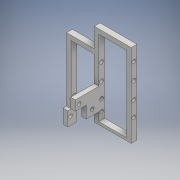
# Autodesk Inventor part: Mounting bracket
Saved by Autodesk Inventor 2017 (Build 210142000, 142)
## iProperties
Created: 2018-11-02
Part Number: Mounting bracket
Material: Generic
Document SubType Name: Modeling
Designer: Usman
Density: 1 g/cm^3
Appearance: Default
Author: Usman
Autodesk Inventor part; units mm, degrees
ref_plane "YZ Plane" through (0, 0, 0) normal (1, 0, 0) x (0, 1, 0)
ref_plane "XZ Plane" through (0, 0, 0) normal (0, 1, 0) x (-1, 0, 0)
ref_plane "XY Plane" through (0, 0, 0) normal (0, 0, 1) x (1, 0, 0)
sketch "Sketch1" plane through (0, 0, 0) normal (0, 1, 0) x (-1, 0, 0)
  line L0 (0, 0) -> (-30, 0)
  line L1 (-30, 0) -> (-30, -80)
  line L2 (0, 0) -> (0, -21)
  line L3 (0, -21) -> (30, -21)
  line L4 (30, -21) -> (30, -80)
  line L5 (30, -80) -> (30, -112)
  line L6 (30, -112) -> (8.74, -112)
  line L7 (8.74, -112) -> (8.74, -80)
  line L8 (8.74, -80) -> (-30, -80)
  line L9 (-35, 5) -> (-35, -85)
  line L10 (-35, -85) -> (3.74, -85)
  line L11 (3.74, -85) -> (3.74, -117)
  line L12 (-35, 5) -> (5, 5)
  line L13 (5, 5) -> (5, -16)
  line L14 (5, -16) -> (35, -16)
  line L15 (35, -16) -> (35, -117)
  line L16 (35, -117) -> (3.74, -117)
  line L17 (0, -21) -> (5, -21)
  line L18 (0, -21) -> (5, -21)
  line L19 (5, -21) -> (5, -80)
  line L20 (0, -21) -> (0, -80)
  dimension "d0" = 30
  dimension "d2" = 21
  dimension "d3" = 30
  dimension "d4" = 59
  dimension "d5" = 32
  dimension "d6" = 21.26
  dimension "d9" = 90
  dimension "d10" = 38.74
  dimension "d11" = 32
  dimension "d12" = 40
  dimension "d13" = 21
  dimension "d14" = 30
  constraints: 42 end point, 13 perpendicular, 4 point on line, 2 horizontal, 2 vertical, 1 collinear, 1 parallel
  measures "d0" distance of L0.start L0.end
  measures "d2" distance of L0.start L2.end
  measures "d3" distance of L2.end L3.end
  measures "d4" distance of L3.end L4.end
  measures "d5" distance of L4.end L5.end
  measures "d6" distance of L5.end L6.end
  measures "d9" distance of L9.start L9.end
  measures "d10" distance of L9.end L10.end
  measures "d11" distance of L10.end L11.end
  measures "d12" distance of L9.start L12.end
  measures "d13" distance of L12.end L13.end
  measures "d14" distance of L13.end L14.end
extrude "Extrusion1" add sketch "Sketch1" along normal blind 16 contours L3 L19 L8 L20 | L12 L13 L14 L15 L16 L11 L10 L9
sketch "Sketch2" plane through (0, 16, 0) normal (0, 1, 0) x (1, 0, 0)
  line L0 (35, -5) -> (35, 85) projected
  line L1 (35, 85) -> (-46.5269, 85)
  line L2 (-46.5269, 85) -> (-46.5269, 122.3541)
  line L3 (-46.5269, 122.3541) -> (35, 122.3541)
  line L4 (35, 122.3541) -> (35, 85)
  point P0 (0, 0)
  constraints: 8 end point, 2 parallel, 1 horizontal, 1 perpendicular
extrude "Extrusion2" cut sketch "Sketch2" against normal blind 16
sketch "Sketch3" plane through (0, 16, 0) normal (0, 1, 0) x (1, 0, 0)
  line L0 (-5, 21) -> (-5, 80) projected
  line L1 (-5, 78.0031) -> (-14.0245, 78.0031)
  line L2 (-14.0245, 78.0031) -> (-14.0245, 94.0311)
  line L3 (-14.0245, 94.0311) -> (-5, 94.0311)
  line L4 (-5, 94.0311) -> (-5, 78.0031)
  point P0 (0, 0)
  constraints: 8 end point, 2 parallel, 1 horizontal, 1 perpendicular, 1 point on line
extrude "Extrusion3" cut sketch "Sketch3" against normal blind 16
sketch "Sketch5" plane through (35, 0, 5) normal (1, 0, 0) x (0, 0, -1)
  line L0 (0, 0) -> (90, 0) projected
  line L1 (0, 0) -> (9.5, 0)
  line L2 (9.5, 0) -> (9.5, 6.622)
  line L3 (9.5, 0) -> (14.5, 0)
  line L4 (14.5, 0) -> (14.5, 6.622)
  circle A0 centre (14.5, 6.622) radius 2.083
  point P0 (5, 0)
  dimension "d21" = 9.5
  dimension "d23" = 5
  dimension "d24" = 6.622
  dimension "d25" = 4.166
  constraints: 8 end point, 2 perpendicular, 2 point on line, 1 centre point, 1 coincident
  measures "d21" distance of L0.start L1.end
  measures "d23" distance of L1.end L3.end
  measures "d24" distance of L3.end L4.end
  measures "d25" diameter of A0
extrude "Extrusion4" cut sketch "Sketch5" against normal blind 16
sketch "Sketch6" plane through (0, 0, -80) normal (1, 0, 0) x (0, 0, -1)
  circle A0 centre (-70.5, 6.622) radius 2.083 projected
  line L0 (-70.5, 6.622) -> (-52.5, 6.622)
  circle A1 centre (-52.5, 6.622) radius 2.0828
  point P0 (-80, 0)
  dimension "d29" = 18
  dimension "d30" = 4.1656
  constraints: 2 end point, 1 centre point, 1 coincident, 1 horizontal
  measures "d29" distance of L0.start L0.end
  measures "d30" diameter of A1
extrude "Extrusion5" cut sketch "Sketch6" along normal blind 50 and the other way blind 25 contours A1
sketch "Sketch7" plane through (35, 0, 5) normal (1, 0, 0) x (0, 0, -1)
  circle A0 centre (32.5, 6.622) radius 2.0828 projected
  line L0 (32.5, 6.622) -> (50.5, 6.622)
  line L1 (50.5, 6.622) -> (67, 6.622)
  circle A1 centre (50.5, 6.622) radius 2.0828
  circle A2 centre (67, 6.622) radius 2.0828
  point P0 (5, 0)
  dimension "d37" = 18
  dimension "d38" = 16.5
  dimension "d39" = 4.1656
  dimension "d40" = 4.1656
  constraints: 4 end point, 2 centre point, 2 coincident, 1 horizontal, 1 point on line
  measures "d37" distance of L0.start L0.end
  measures "d38" distance of L0.end L1.end
  measures "d39" diameter of A1
  measures "d40" diameter of A2
extrude "Extrusion6" cut sketch "Sketch7" against normal blind 50 contours A1 L1 L0 | L0 L1 A1 | A2
sketch "Sketch9" plane through (0, 0, -80) normal (1, 0, 0) x (0, 0, -1)
  circle A0 centre (-18, 6.622) radius 2.0828 projected
  line L0 (-18, 6.622) -> (-6, 6.622)
  circle A1 centre (-6, 6.622) radius 2.0828
  point P0 (-80, 0)
  dimension "d43" = 12
  dimension "d44" = 4.1656
  constraints: 2 end point, 1 centre point, 1 coincident, 1 horizontal
  measures "d43" distance of L0.start L0.end
  measures "d44" diameter of A1
extrude "Extrusion7" cut sketch "Sketch9" against normal blind 10 contours A1
sketch "Sketch10" plane through (0, 0, 0) normal (0, -1, 0) x (1, 0, 0)
  line L0 (0, -80.0219) -> (8.5, -80.0219)
  line L1 (8.5, -80.0219) -> (8.5, -82.0219)
  line L2 (8.5, -82.0219) -> (0, -82.0219)
  line L3 (0, -82.0219) -> (0, -80.0219)
  line L4 (8.5, -80.0219) -> (11.5, -80.0219)
  line L5 (11.5, -80.0219) -> (11.5, -82.0219)
  line L6 (11.5, -82.0219) -> (8.5, -82.0219)
  line L7 (8.5, -82.0219) -> (8.5, -80.0219)
  line L8 (8.5, -80.0219) -> (11.5, -80.0219)
  line L9 (11.5, -80.0219) -> (11.5, -75.0982)
  line L10 (11.5, -75.0982) -> (8.5, -75.0982)
  line L11 (8.5, -75.0982) -> (8.5, -80.0219)
  line L12 (30, 0) -> (30, -80) projected
  line L13 (30, -80) -> (21.5, -80)
  line L14 (21.5, -80) -> (21.5, -82.0219)
  line L15 (21.5, -82.0219) -> (30, -82.0219)
  line L16 (30, -82.0219) -> (30, -80)
  line L17 (21.5, -82.0219) -> (17, -82.0219)
  line L18 (17, -82.0219) -> (17, -71.2839)
  line L19 (17, -71.2839) -> (21.5, -71.2839)
  line L20 (21.5, -71.2839) -> (21.5, -82.0219)
  point P0 (0, 0)
  dimension "d47" = 8.5
  dimension "d48" = 2
  dimension "d49" = 3
  dimension "d50" = 8.5
  dimension "d51" = 4.5
  constraints: 40 end point, 10 parallel, 5 horizontal, 5 perpendicular
  measures "d47" distance of L1.end L2.end
  measures "d48" distance of L0.end L1.end
  measures "d49" distance of L5.end L6.end
  measures "d50" distance of L15.end L14.end
  measures "d51" distance of L18.end L19.end
extrude "Extrusion8" cut sketch "Sketch10" against normal blind 100 contours L14 L17 L18 L19 L20
sketch "Sketch11" plane through (0, 16, 0) normal (0, 1, 0) x (1, 0, 0)
  line L0 (-38.388, 86.2009) -> (-26.8829, 86.2009)
  line L1 (-26.8829, 86.2009) -> (-26.8829, 63.045)
  line L2 (-26.8829, 63.045) -> (-38.388, 63.045)
  line L3 (-38.388, 63.045) -> (-38.388, 86.2009)
  point P0 (0, 0)
  constraints: 8 end point, 2 parallel, 1 horizontal, 1 perpendicular
extrude "Extrusion9" cut sketch "Sketch11" against normal blind 100
sketch "Sketch12" plane through (0, 0, 0) normal (0, -1, 0) x (1, 0, 0)
  line L0 (17, -80) -> (0, -80) projected
  line L1 (17, -82.0219) -> (17, -80)
  line L2 (17, -80) -> (0, -80)
  line L3 (0, -80) -> (0, -82.0219)
  line L4 (21.5, -82.0219) -> (17, -82.0219) projected
  line L5 (0, -82.0219) -> (17, -82.0219)
  point P0 (0, 0)
  constraints: 8 end point, 2 collinear, 2 perpendicular
extrude "Extrusion10" cut sketch "Sketch12" against normal blind 16000
sketch "Sketch13" plane through (0, 0, 0) normal (0, -1, 0) x (1, 0, 0)
  line L0 (30, -80) -> (21.5, -80) projected
  line L1 (30, -80) -> (21.5, -80)
  line L2 (21.5, -80) -> (21.5, -82.0219) projected
  line L3 (21.5, -80) -> (21.5, -82.0219)
  line L4 (21.5, -82.0219) -> (30, -82.0219)
  line L5 (30, -82.0219) -> (30, -80)
  point P0 (0, 0)
  constraints: 8 end point, 2 collinear, 2 perpendicular
extrude "Extrusion11" cut sketch "Sketch13" against normal blind 16000
sketch "Sketch14" plane through (0, 0, 0) normal (0, -1, 0) x (1, 0, 0)
  line L0 (-37.2661, -60.1404) -> (-28.1164, -60.1404)
  line L1 (-28.1164, -60.1404) -> (-28.1164, -64.2388)
  line L2 (-28.1164, -64.2388) -> (-37.2661, -64.2388)
  line L3 (-37.2661, -64.2388) -> (-37.2661, -60.1404)
  point P0 (0, 0)
  constraints: 8 end point, 2 parallel, 1 horizontal, 1 perpendicular
extrude "Extrusion12" cut sketch "Sketch14" against normal blind 10000
sketch "Sketch15" plane through (0, 0, 0) normal (0, -1, 0) x (1, 0, 0)
  line L0 (-5, -85) -> (-5, -21) projected
  line L1 (0, 0) -> (0, -82.0219) projected
  line L2 (-5, -47.0884) -> (0, -47.0884)
  line L3 (0, -47.0884) -> (0, -60.3662)
  line L4 (0, -60.3662) -> (-5, -60.3662)
  line L5 (-5, -60.3662) -> (-5, -47.0884)
  constraints: 8 end point, 2 parallel, 2 point on line, 1 horizontal, 1 perpendicular
extrude "Extrusion13" add sketch "Sketch15" along normal blind 10
sketch "Sketch16" plane through (0, -10, 0) normal (0, -1, 0) x (1, 0, 0)
  line L0 (0, -47.0884) -> (-5, -47.0884) projected
  line L1 (0, 0) -> (0, -82.0219) projected
  line L2 (-5, -47.0884) -> (0, -47.0884)
  line L3 (0, -47.0884) -> (0, -53.8884)
  line L4 (0, -53.8884) -> (-5, -53.8884)
  line L5 (-5, -53.8884) -> (-5, -47.0884)
  line L6 (0, -82.0219) -> (0, -60.3662) projected
  line L7 (-5, -53.8884) -> (0, -53.8884)
  line L8 (0, -53.8884) -> (0, -68.0271)
  line L9 (0, -68.0271) -> (-5, -68.0271)
  line L10 (-5, -68.0271) -> (-5, -53.8884)
  dimension "d64" = 6.8
  constraints: 16 end point, 4 parallel, 2 horizontal, 2 perpendicular, 2 point on line
  measures "d64" distance of L2.end L3.end
extrude "Extrusion14" add sketch "Sketch16" along normal mid plane 20 contours L1 L9 L10 L4
sketch "Sketch17" plane through (0, -10, 0) normal (0, -1, 0) x (1, 0, 0)
  line L0 (0, -47.0884) -> (-5, -47.0884) projected
  line L1 (0, -53.8884) -> (0, -47.0884) projected
  line L2 (-5, -47.0884) -> (0, -47.0884)
  line L3 (0, -47.0884) -> (0, -53.8884)
  line L4 (0, -53.8884) -> (-5, -53.8884)
  line L5 (-5, -53.8884) -> (-5, -47.0884)
  point P0 (0, 0)
  constraints: 8 end point, 2 parallel, 1 horizontal, 1 perpendicular
extrude "Extrusion15" cut sketch "Sketch17" against normal blind 10
sketch "Sketch18" plane through (0, -20, 0) normal (0, -1, 0) x (1, 0, 0)
  line L0 (-5, -53.8884) -> (-5, -68.0271) projected
  line L1 (0, -71.9172) -> (0, -76.0828) projected
  line L2 (-5, -68.0271) -> (0, -68.0271)
  line L3 (0, -68.0271) -> (0, -76.0828)
  line L4 (0, -76.0828) -> (-5, -76.0828)
  line L5 (-5, -76.0828) -> (-5, -68.0271)
  point P0 (0, 0)
  constraints: 8 end point, 2 parallel, 1 horizontal, 1 perpendicular
extrude "Extrusion16" add sketch "Sketch18" against normal blind 20
sketch "Sketch19" plane through (0, -20, 0) normal (0, -1, 0) x (1, 0, 0)
  line L0 (-5, -76.0828) -> (-5, -85) projected
  line L1 (0, -53.8884) -> (0, -76.0828) projected
  line L2 (-5, -76.0828) -> (0, -76.0828)
  line L3 (0, -76.0828) -> (0, -70.4113)
  line L4 (0, -70.4113) -> (-5, -70.4113)
  line L5 (-5, -70.4113) -> (-5, -76.0828)
  point P0 (0, 0)
  constraints: 8 end point, 2 parallel, 1 horizontal, 1 perpendicular, 1 point on line
extrude "Extrusion17" cut sketch "Sketch19" against normal blind 10
sketch "Sketch20" plane through (-5, 0, -21) normal (-1, 0, 0) x (0, 0, 1)
  line L0 (-55.0828, -10) -> (-49.4113, -10) projected
  line L1 (21, 0) -> (-61.0219, 0) projected
  line L2 (-55.0828, -10) -> (-51.8224, -10)
  line L3 (-51.8224, -10) -> (-51.8224, 0)
  line L4 (-51.8224, 0) -> (-55.0828, 0)
  line L5 (-55.0828, 0) -> (-55.0828, -10)
  constraints: 8 end point, 2 parallel, 1 horizontal, 1 perpendicular, 1 point on line
extrude "Extrusion18" cut sketch "Sketch20" against normal blind 10
sketch "Sketch21" plane through (-5, 0, -21) normal (-1, 0, 0) x (0, 0, 1)
  circle A0 centre (-53, 6.622) radius 2.0828 projected
  line L0 (-53, 6.622) -> (-45.8284, -3.6161)
  circle A1 centre (-45.8284, -3.6161) radius 2.0828
  point P0 (21, 0)
  dimension "d75" = 12.5
  dimension "d76" = 4.1656
  constraints: 2 end point, 1 centre point, 1 coincident
  measures "d75" distance of L0.start L0.end
  measures "d76" diameter of A1
extrude "Extrusion19" cut sketch "Sketch21" against normal blind 20 contours A1
sketch "Sketch22" plane through (-5, 0, -21) normal (-1, 0, 0) x (0, 0, 1)
  circle A0 centre (-45.8284, -3.6161) radius 2.0828 projected
  line L0 (-45.8284, -3.6161) -> (-33.8473, -17.7123)
  circle A1 centre (-33.8473, -17.7123) radius 2.0828
  point P0 (21, 0)
  dimension "d79" = 18.5
  dimension "d86" = 4.1656
  constraints: 2 end point, 1 centre point, 1 coincident
  measures "d79" distance of L0.start L0.end
  measures "d86" diameter of A1
sketch "Sketch23" plane through (0, 0, 0) normal (0, -1, 0) x (1, 0, 0)
  line L0 (-5, -53.8884) -> (0, -53.8884)
  line L1 (0, -53.8884) -> (0, -48.8884)
  line L2 (0, -48.8884) -> (-5, -48.8884)
  line L3 (-5, -48.8884) -> (-5, -53.8884)
  point P0 (0, 0)
  dimension "d80" = 5
  dimension "d81" = 5
  constraints: 8 end point, 2 parallel, 1 horizontal, 1 perpendicular
  measures "d80" distance of L2.end L1.end
  measures "d81" distance of L1.end L0.end
extrude "Extrusion20" add sketch "Sketch23" along normal blind 24
sketch "Sketch24" plane through (0, -20, 0) normal (0, -1, 0) x (1, 0, 0)
  line L0 (0, -53.8884) -> (-5, -53.8884) projected
  line L1 (-5, -70.4113) -> (0, -70.4113) projected
  line L2 (-5, -53.8884) -> (0, -53.8884)
  line L3 (0, -53.8884) -> (0, -70.4113)
  line L4 (0, -70.4113) -> (-5, -70.4113)
  line L5 (-5, -70.4113) -> (-5, -53.8884)
  point P0 (0, 0)
  constraints: 8 end point, 2 parallel, 1 horizontal, 1 perpendicular
extrude "Extrusion21" add sketch "Sketch24" along normal blind 4
extrude "Extrusion22" cut sketch "Sketch22" against normal blind 10 contours A1
sketch "Sketch25" plane through (-5, 0, -21) normal (-1, 0, 0) x (0, 0, 1)
  line L0 (-49.4113, -10) -> (-49.4113, -24) projected
  line L1 (-27.8884, 0) -> (-27.8884, -24) projected
  line L2 (-49.4113, -24) -> (-27.8884, -24)
  line L3 (-27.8884, -24) -> (-27.8884, -21.7301)
  line L4 (-27.8884, -21.7301) -> (-49.4113, -21.7301)
  line L5 (-49.4113, -21.7301) -> (-49.4113, -24)
  point P0 (21, 0)
  constraints: 8 end point, 2 parallel, 1 horizontal, 1 perpendicular, 1 point on line
extrude "Extrusion23" cut sketch "Sketch25" against normal blind 10
sketch "Sketch26" plane through (0, 16, 0) normal (0, 1, 0) x (1, 0, 0)
  line L0 (-35, 60.1404) -> (-30, 60.1404) projected
  line L1 (-35, 60.1404) -> (-30, 60.1404)
  line L2 (-30, 60.1404) -> (-30, 100.1404)
  line L3 (-30, 100.1404) -> (-35, 100.1404)
  line L4 (-35, 100.1404) -> (-35, 60.1404)
  point P0 (0, 0)
  dimension "d91" = 40
  constraints: 8 end point, 2 parallel, 1 horizontal, 1 perpendicular
  measures "d91" distance of L2.end L1.end
extrude "Extrusion24" add sketch "Sketch26" against normal blind 16
sketch "Sketch29" plane through (35, 0, 5) normal (1, 0, 0) x (0, 0, -1)
  line L0 (0, 16) -> (90, 16) projected
  line L1 (105.1404, 16) -> (105.1404, 0) projected
  line L2 (0, 16) -> (105.1404, 16)
  line L3 (105.1404, 16) -> (105.1404, 10)
  line L4 (105.1404, 10) -> (0, 10)
  line L5 (0, 10) -> (0, 16)
  line L6 (0, 0) -> (90, 0) projected
  point P0 (5, 0)
  dimension "d101" = 10
  constraints: 8 end point, 2 parallel, 1 horizontal, 1 perpendicular, 1 point on line
  measures "d101" distance between parallel lines of L6 L4
extrude "Extrusion27" cut sketch "Sketch29" against normal blind 70
sketch "Sketch30" plane through (-35, 0, -100.1404) normal (-1, 0, 0) x (0, 0, 1)
  line L0 (105.1404, 0) -> (15.1404, 0) projected
  line L1 (105.1404, 0) -> (51.2521, 0)
  line L2 (51.2521, 0) -> (51.2521, 3.75)
  line L3 (51.2521, 3.75) -> (105.1404, 3.75)
  line L4 (105.1404, 3.75) -> (105.1404, 0)
  line L5 (51.2521, 0) -> (51.2521, -21.7301) projected
  point P0 (100.1404, 0)
  dimension "d104" = 3.75
  dimension "d115" = 0
  constraints: 8 end point, 2 parallel, 1 horizontal, 1 perpendicular
  measures "d104" distance between parallel lines of L0 L3
  measures "d115" distance between parallel lines of L2 L5
extrude "Extrusion28" cut sketch "Sketch30" against normal blind 70
sketch "Sketch31" plane through (35, 0, -85) normal (1, 0, 0) x (0, 0, -1)
  line L0 (-36.1116, 3.75) -> (-64, 3.75) projected
  line L1 (-36.1116, 0) -> (0, 0) projected
  line L2 (-36.1116, 3.75) -> (0, 3.75)
  line L3 (0, 3.75) -> (0, 0)
  line L4 (0, 0) -> (-36.1116, 0)
  line L5 (-36.1116, 0) -> (-36.1116, 3.75)
  point P0 (-85, 0)
  constraints: 8 end point, 2 parallel, 1 horizontal, 1 perpendicular
extrude "Extrusion29" cut sketch "Sketch31" against normal blind 30
sketch "Sketch32" plane through (35, 10, -85) normal (0, 0, -1) x (-1, 0, 0)
  line L0 (40, -6.25) -> (35, -6.25) projected
  line L1 (29.9543, -10) -> (40, -10)
  line L2 (40, -10) -> (40, -6.25)
  line L3 (40, -6.25) -> (29.9543, -6.25)
  line L4 (29.9543, -6.25) -> (29.9543, -10)
  point P0 (35, -10)
  constraints: 8 end point, 2 parallel, 1 horizontal, 1 perpendicular
extrude "Extrusion30" cut sketch "Sketch32" against normal blind 12.2
sketch "Sketch33" plane through (-5, -10, -72.8224) normal (-1, 0, 0) x (0, 0, 1)
  line L0 (2.4111, 0) -> (2.4111, -11.7301) projected
  line L1 (23.934, -11.7301) -> (2.4111, -11.7301) projected
  line L2 (2.4111, 0) -> (13.1725, 0)
  line L3 (13.1725, 0) -> (13.1725, -11.7301)
  line L4 (13.1725, -11.7301) -> (2.4111, -11.7301)
  line L5 (2.4111, -11.7301) -> (2.4111, 0)
  point P0 (72.8224, 10)
  constraints: 8 end point, 2 parallel, 1 horizontal, 1 midpoint, 1 perpendicular
extrude "Extrusion31" cut sketch "Sketch33" against normal blind 12.2
sketch "Sketch35" plane through (-35, 0, -100.1404) normal (-1, 0, 0) x (0, 0, 1)
  line L0 (18.1185, 3.75) -> (100.1404, 3.75) projected
  line L1 (52.6043, 3.75) -> (49.8728, 3.75)
  line L2 (49.8728, 3.75) -> (49.8728, 0)
  line L3 (49.8728, 0) -> (52.6043, 0)
  line L4 (52.6043, 0) -> (52.6043, 3.75)
  point P0 (100.1404, 0)
  constraints: 8 end point, 2 parallel, 1 horizontal, 1 perpendicular, 1 point on line
extrude "Extrusion33" cut sketch "Sketch35" against normal blind 5
sketch "Sketch36" plane through (-35, 0, -100.1404) normal (-1, 0, 0) x (0, 0, 1)
  circle A0 centre (26.141, 6.622) radius 2.083
  line L0 (0, 10) -> (0, 0) projected
  line L1 (49.8728, 3.75) -> (84.1404, 3.75) projected
  point P0 (100.1404, 0)
  point P1 (15.1404, 3.75)
  dimension "d118" = 4.166
  dimension "d119" = 26.141
  dimension "d120" = 2.872
  constraints: 1 centre point
  measures "d118" diameter of A0
  measures "d119" distance from line of L0 A0.centre
  measures "d120" distance from line of A0.centre L1
extrude "Extrusion34" cut sketch "Sketch36" against normal blind 10
sketch "Sketch37" plane through (-35, 0, -100.1404) normal (-1, 0, 0) x (0, 0, 1)
  line L0 (49.8728, 0) -> (49.8728, 3.75) projected
  line L1 (15.1404, 3.75) -> (15.1404, 10) projected
  line L2 (49.8728, 0) -> (15.1404, 0)
  line L3 (15.1404, 0) -> (15.1404, 3.75)
  line L4 (15.1404, 3.75) -> (49.8728, 3.75)
  line L5 (49.8728, 3.75) -> (49.8728, 0)
  point P0 (100.1404, 0)
  constraints: 8 end point, 2 parallel, 1 horizontal, 1 perpendicular
extrude "Extrusion35" cut sketch "Sketch37" against normal blind 5
sketch "Sketch39" plane through (-35, 0, -100.1404) normal (-1, 0, 0) x (0, 0, 1)
  circle A0 centre (8.534, 2.88) radius 2.083
  line L0 (0, 10) -> (0, 0) projected
  line L1 (0, 0) -> (15.1404, 0) projected
  point P0 (100.1404, 0)
  dimension "d131" = 4.166
  dimension "d132" = 6.451
  dimension "d133" = 2.88
  constraints: 1 centre point
  measures "d131" diameter of A0
  measures "d132" distance edge to line of A0 L0
  measures "d133" distance from line of L1 A0.centre
extrude "Extrusion37" cut sketch "Sketch39" against normal blind 5
body "Solid1"
